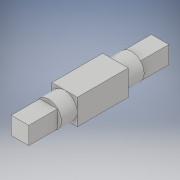
# Autodesk Inventor part: GearAxis
Saved by Autodesk Inventor 2017 (Build 210142000, 142)
## iProperties
Created: 2020-04-04
Part Number: GearAxis
Material: Generic
Document SubType Name: Modeling
Designer: LaNave
Density: 1 g/cm^3
Appearance: Default
Mass: 1.37765 g
Surface Area: 8.99327 cm^2
Volume: 1.37765 cm^3
Author: LaNave
## iProperties of the stored document gear2-shaft_3DPrint.ipt
Created: 2021-01-25
Part Number: gear2-shaft_3DPrint
Material: Generic
Document SubType Name: Modeling
Designer: agustin
Density: 1 g/cm^3
Appearance: Default
Author: agustin
Autodesk Inventor part; units mm, degrees
ref_plane "YZ Plane" through (0, 0, 0) normal (1, 0, 0) x (0, 1, 0)
ref_plane "XZ Plane" through (0, 0, 0) normal (0, 1, 0) x (-1, 0, 0)
ref_plane "XY Plane" through (0, 0, 0) normal (0, 0, 1) x (1, 0, 0)
sketch "Sketch1" plane through (0, 0, 0) normal (0, 0, 1) x (1, 0, 0)
  circle A0 centre (0, 0) radius 4
  line L0 (4, 0) -> (2, -3.4641)
  line L1 (2, -3.4641) -> (-2, -3.4641)
  line L2 (-2, -3.4641) -> (-4, 0)
  line L3 (-4, 0) -> (-2, 3.4641)
  line L4 (-2, 3.4641) -> (2, 3.4641)
  line L5 (2, 3.4641) -> (4, 0)
  dimension "d0" = 8
  constraints: 12 end point, 2 coincident, 1 horizontal alignment, 15 other
extrude "Extrusion1" add sketch "Sketch1" against normal blind 5
sketch "Sketch2" plane through (0, 0, -5) normal (0, 0, -1) x (-1, 0, 0)
  circle A0 centre (0, 0) radius 4 projected
  line L0 (-4, 4) -> (4, 4)
  line L1 (4, 4) -> (4, -4)
  line L2 (4, -4) -> (-4, -4)
  line L3 (-4, -4) -> (-4, 4)
  point P0 (-4, 0)
  constraints: 8 end point, 1 horizontal alignment, 1 midpoint, 10 other
extrude "Extrusion2" add sketch "Sketch2" along normal blind 8
sketch "Sketch3" plane through (0, 0, 0) normal (0, 0, 1) x (1, 0, 0)
  line L0 (4, -2.3094) -> (0, -4.6188) projected
  line L1 (-2.75, -2.75) -> (-2.75, 2.75)
  line L2 (-2.75, 2.75) -> (2.75, 2.75)
  line L3 (2.75, 2.75) -> (2.75, -2.75)
  line L4 (2.75, -2.75) -> (-2.75, -2.75)
  point P0 (0, 0)
  point P1 (0, -2.75)
  dimension "d7" = 5.5
  dimension "d8" = 5.5
  constraints: 8 end point, 1 midpoint, 9 other
  measures "d7" distance of L2.end L3.end
  measures "d8" distance of L3.end L1.start
extrude "Extrusion3" add sketch "Sketch3" along normal blind 9
mirror "Mirror1" about plane through (0, 0, -13) normal (0, 0, -1) of "Extrusion1", "Extrusion2", "Extrusion3"
scale "Scale1" factors (0.5, 0.5, 0.5) then translate (0, 2, -6.5) bodies 1
body "Solid1"
